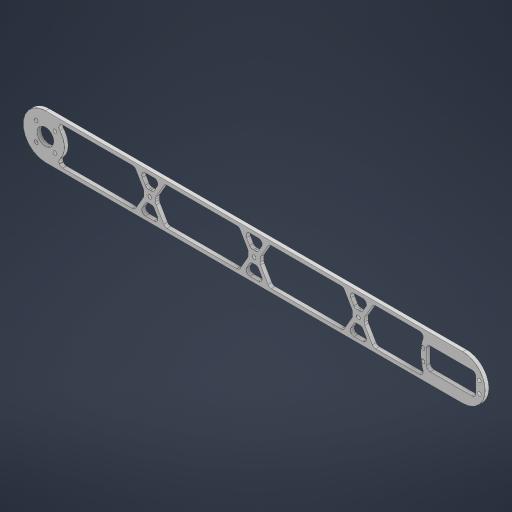
# Autodesk Inventor part: Arm3rdLinkServo
Saved by Autodesk Inventor 2023 (Build 270158000, 158)
## iProperties
Created: 2023-12-24
Part Number: Arm3rdLinkServo
Material: Generic
Document SubType Name: Modeling
Designer: kelle
Density: 1 g/cm^3
Appearance: Default
Author: kelle
Autodesk Inventor part; units mm, degrees
ref_plane "YZ Plane" through (0, 0, 0) normal (1, 0, 0) x (0, 1, 0)
ref_plane "XZ Plane" through (0, 0, 0) normal (0, 1, 0) x (-1, 0, 0)
ref_plane "XY Plane" through (0, 0, 0) normal (0, 0, 1) x (1, 0, 0)
sketch "Sketch1" plane through (0, 0, 0) normal (0, 0, 1) x (1, 0, 0)
  line L0 (177.8, 0) -> (-177.8, 0) construction
  line L1 (177.8, 19.05) -> (-177.8, 19.05)
  line L2 (-177.8, -19.05) -> (177.8, -19.05)
  arc A0 (177.8, -19.05) -> (177.8, 19.05) centre (177.8, 0) ccw
  arc A1 (-177.8, 19.05) -> (-177.8, -19.05) centre (-177.8, 0) ccw
  circle A2 centre (-177.8, 0) radius 7
  line L3 (-185.8, -8) -> (-169.8, -8) construction
  line L4 (-169.8, -8) -> (-169.8, 8) construction
  line L5 (-169.8, 8) -> (-185.8, 8) construction
  line L6 (-185.8, 8) -> (-185.8, -8) construction
  line L7 (-185.8, -8) -> (-169.8, 8) construction
  line L8 (-169.8, -8) -> (-185.8, 8) construction
  circle A3 centre (-185.8, 8) radius 1.5875
  circle A4 centre (-169.8, 8) radius 1.5875
  circle A5 centre (-185.8, -8) radius 1.5875
  circle A6 centre (-169.8, -8) radius 1.5875
  circle A7 centre (0, 0) radius 2
  circle A8 centre (-88.9, 0) radius 2
  circle A9 centre (88.9, 0) radius 2
  circle A10 centre (0, 0) radius 2
  circle A11 centre (177.8, 0) radius 3
  line L9 (177.8, 0) -> (192, 0) construction
  line L10 (192, 0) -> (192, 4.95) construction
  circle A12 centre (192, 4.95) radius 1.5875
  circle A13 centre (144, 4.95) radius 1.5875
  circle A14 centre (192, -4.95) radius 1.5875
  circle A15 centre (144, -4.95) radius 1.5875
  line L11 (192, 4.95) -> (189, 4.95) construction
  line L12 (189, 9.525) -> (147, 9.525)
  line L13 (147, 9.525) -> (147, -9.525)
  line L14 (189, -9.525) -> (189, 9.525)
  line L15 (147, -9.525) -> (189, -9.525)
  dimension "d0" = 177.8
  dimension "d1" = 38.1
  dimension "d2" = 14
  dimension "d3" = 16
  dimension "d4" = 16
  dimension "d5" = 3.175
  dimension "d8" = 16
  dimension "d11" = 16
  dimension "d14" = 4
  dimension "d17" = 88.9
  dimension "d20" = 88.9
  dimension "d23" = 6
  dimension "d24" = 14.2
  dimension "d25" = 4.95
  dimension "d27" = 3.175
  dimension "d31" = 48
  dimension "d34" = 9.9
  dimension "d37" = 3
  dimension "d38" = 42
  dimension "d39" = 9.525
  dimension "d40" = 19.05
  dimension "d41" = 42
  dimension "d60" = 3
  constraints: 34 end point, 16 centre point, 9 horizontal, 5 coincident, 4 point on circle, 4 tangent, 4 vertical, 3 midpoint, 3 parallel, 1 perpendicular, 18 other
  measures "d0" distance of point (0, 0) L0.end
  measures "d1" diameter of A1
  measures "d2" diameter of A2
  measures "d3" distance of L3.start L3.end
  measures "d4" distance of L4.end L3.end
  measures "d5" diameter of A3
  measures "d8" distance of A3.centre A4.centre
  measures "d11" distance of A3.centre A5.centre
  measures "d14" diameter of A7
  measures "d17" distance of A7.centre A8.centre
  measures "d20" distance of A7.centre A9.centre
  measures "d23" diameter of A11
  measures "d24" distance of L9.start L9.end
  measures "d25" distance of L9.end L10.end
  measures "d27" diameter of A12
  measures "d31" distance of L11.start A13.centre
  measures "d34" distance of L11.start A14.centre
  measures "d37" distance of L11.start L11.end
  measures "d38" distance of L12.start L12.end
  measures "d39" distance between parallel lines of L12 L0
  measures "d40" distance of L12.end L13.end
  measures "d41" distance of L13.end L14.start
  measures "d60" distance from line of L10.end L14
extrude "Extrusion1" add sketch "Sketch1" along normal blind 3.175 contours A0 L2 A1 L1
sketch "Sketch4" plane through (0, 0, 3.175) normal (0, 0, 1) x (1, 0, 0)
  arc A0 (-177.8, 19.05) -> (-177.8, -19.05) centre (-177.8, 0) ccw
  line L0 (-177.8, -19.05) -> (177.8, -19.05)
  arc A1 (177.8, -19.05) -> (177.8, 19.05) centre (177.8, 0) ccw
  line L1 (177.8, 19.05) -> (-177.8, 19.05)
  circle A2 centre (0, 0) radius 2
  circle A3 centre (-88.9, 0) radius 2
  circle A4 centre (88.9, 0) radius 2
  circle A5 centre (144, 4.95) radius 1.5875
  circle A6 centre (144, -4.95) radius 1.5875
  line L2 (189, 9.525) -> (189, -9.525)
  line L3 (189, -9.525) -> (147, -9.525)
  line L4 (147, -9.525) -> (147, 9.525)
  line L5 (147, 9.525) -> (189, 9.525)
  circle A7 centre (192, -4.95) radius 1.5875
  circle A8 centre (192, 4.95) radius 1.5875
  circle A9 centre (-169.8, -8) radius 1.5875
  circle A10 centre (-185.8, -8) radius 1.5875
  circle A11 centre (-169.8, 8) radius 1.5875
  circle A12 centre (-185.8, 8) radius 1.5875
  circle A13 centre (-177.8, 0) radius 7
  circle A14 centre (-177.8, 0) radius 7 construction
  circle A15 centre (-177.8, 0) radius 12.901208 construction
  circle A16 centre (-177.8, 0) radius 16.076208
  circle A17 centre (-88.9, 0) radius 5.175
  circle A18 centre (0, 0) radius 5.175
  circle A19 centre (88.9, 0) radius 5.175
  circle A20 centre (177.8, 0) radius 35.74804
  circle A21 centre (144, -4.95) radius 1.5875 construction
  circle A22 centre (177.8, 0) radius 38.92304 construction
  line L6 (-177.8, 0) -> (-133.35, 0) construction
  line L7 (-177.8, 0) -> (-133.35, 0) construction
  line L8 (-177.8, 0) -> (-155.575, 38.494829)
  line L9 (-155.575, 38.494829) -> (-111.125, 38.494829)
  line L10 (-111.125, 38.494829) -> (-88.9, 0)
  line L11 (-88.9, 0) -> (-111.125, -38.494829)
  line L12 (-111.125, -38.494829) -> (-155.575, -38.494829)
  line L13 (-155.575, -38.494829) -> (-177.8, 0)
  arc A23 (-177.8, 15.875) -> (-177.8, -15.875) centre (-177.8, 0) ccw
  line L14 (-177.8, -15.875) -> (177.8, -15.875)
  arc A24 (177.8, -15.875) -> (177.8, 15.875) centre (177.8, 0) ccw
  line L15 (177.8, 15.875) -> (-177.8, 15.875)
  line L16 (-112.958087, 35.319829) -> (-153.741913, 35.319829)
  line L17 (-153.741913, 35.319829) -> (-174.133826, 0)
  line L18 (-174.133826, 0) -> (-153.741913, -35.319829)
  line L19 (-153.741913, -35.319829) -> (-112.958087, -35.319829)
  line L20 (-112.958087, -35.319829) -> (-92.566174, 0)
  line L21 (-92.566174, 0) -> (-112.958087, 35.319829)
  line L22 (177.8, 19.05) -> (-177.8, 19.05) construction
  line L23 (-88.9, 19.05) -> (-88.9, -19.05) construction
  line L24 (0, 19.05) -> (0, -19.05) construction
  line L25 (0, 0) -> (-22.225, 38.494829)
  line L26 (-66.675, 38.494829) -> (-88.9, 0)
  line L27 (-88.9, 0) -> (-66.675, -38.494829)
  line L28 (-22.225, -38.494829) -> (0, 0)
  line L29 (-24.058087, 35.319829) -> (-3.666174, 0)
  line L30 (-3.666174, 0) -> (-24.058087, -35.319829)
  line L31 (-64.841913, -35.319829) -> (-85.233826, 0)
  line L32 (-85.233826, 0) -> (-64.841913, 35.319829)
  line L33 (177.8, 0) -> (155.575, 38.494829)
  line L34 (111.125, 38.494829) -> (88.9, 0)
  line L35 (88.9, 0) -> (111.125, -38.494829)
  line L36 (155.575, -38.494829) -> (177.8, 0)
  line L37 (153.741913, 35.319829) -> (174.133826, 0)
  line L38 (174.133826, 0) -> (153.741913, -35.319829)
  line L39 (112.958087, -35.319829) -> (92.566174, 0)
  line L40 (92.566174, 0) -> (112.958087, 35.319829)
  line L41 (0, 0) -> (22.225, 38.494829)
  line L42 (24.058087, 35.319829) -> (3.666174, 0)
  line L43 (3.666174, 0) -> (24.058087, -35.319829)
  line L44 (22.225, -38.494829) -> (0, 0)
  line L45 (64.841913, -35.319829) -> (85.233826, 0)
  line L46 (88.9, 0) -> (66.675, -38.494829)
  line L47 (85.233826, 0) -> (64.841913, 35.319829)
  line L48 (66.675, 38.494829) -> (88.9, 0)
  point P0 (79.734564, 15.875)
  point P1 (86.3125, 4.481681)
  point P2 (91.4875, 4.481681)
  point P3 (98.065436, 15.875)
  point P4 (98.065436, -15.875)
  point P5 (91.4875, -4.481681)
  point P6 (86.3125, -4.481681)
  point P7 (79.734564, -15.875)
  point P8 (2.5875, 4.481681)
  point P9 (9.165436, 15.875)
  point P10 (-9.165436, 15.875)
  point P11 (-2.5875, 4.481681)
  point P12 (9.165436, -15.875)
  point P13 (2.5875, -4.481681)
  point P14 (-2.5875, -4.481681)
  point P15 (-9.165436, -15.875)
  point P16 (-79.734564, -15.875)
  point P17 (-86.3125, -4.481681)
  point P18 (-91.4875, -4.481681)
  point P19 (-98.065436, -15.875)
  point P20 (-86.3125, 4.481681)
  point P21 (-79.734564, 15.875)
  point P22 (-98.065436, 15.875)
  point P23 (-91.4875, 4.481681)
  point P24 (93.692912, -1.951568)
  point P25 (101.73161, -15.875)
  point P26 (145.770221, -15.875)
  point P27 (145.770221, 15.875)
  point P28 (101.73161, 15.875)
  point P29 (93.692912, 1.951568)
  point P30 (76.06839, -15.875)
  point P31 (84.107088, -1.951568)
  point P32 (84.107088, 1.951568)
  point P33 (76.06839, 15.875)
  point P34 (12.83161, 15.875)
  point P35 (4.792912, 1.951568)
  point P36 (4.792912, -1.951568)
  point P37 (12.83161, -15.875)
  point P38 (-76.06839, 15.875)
  point P39 (-84.107088, 1.951568)
  point P40 (-84.107088, -1.951568)
  point P41 (-76.06839, -15.875)
  point P42 (-12.83161, -15.875)
  point P43 (-4.792912, -1.951568)
  point P44 (-4.792912, 1.951568)
  point P45 (-12.83161, 15.875)
  point P46 (-93.692912, 1.951568)
  point P47 (-101.73161, 15.875)
  point P48 (-164.96839, 15.875)
  point P49 (-167.170587, 12.060683)
  point P50 (-167.170587, -12.060683)
  point P51 (-164.96839, -15.875)
  point P52 (-101.73161, -15.875)
  point P53 (-93.692912, -1.951568)
  dimension "d61" = 3.175
  dimension "d62" = 3.175
  dimension "d63" = 3.175
  dimension "d64" = 3.175
  dimension "d65" = 3.175
  dimension "d66" = 44.45
  dimension "d67" = 0
  dimension "d68" = 3.175
  dimension "d69" = 3.175
  constraints: 84 end point, 33 symmetric about line, 9 centre point, 4 point on circle, 3 coincident, 2 horizontal, 2 midpoint, 2 point on line, 2 tangent, 1 collinear, 1 perpendicular, 21 other
  measures "d61" radial gap between concentric circles of A15 A16
  measures "d62" radial gap between concentric circles of A3 A17
  measures "d63" radial gap between concentric circles of A2 A18
  measures "d64" radial gap between concentric circles of A4 A19
  measures "d65" radial gap between concentric circles of A20 A22
  measures "d66" distance of L6.start L6.end
  measures "d67" distance between parallel lines of L6 L7
  measures "d68" distance between parallel lines of L1 L15
  measures "d69" distance between parallel lines of L9 L16
extrude "Extrusion4" cut sketch "Sketch4" against normal through all contours L15 L21 A17 L20 L14 L18 A16 L17 | L15 L26 A17 L10 | L11 A17 L27 L14 | L15 L29 A18 L30 L14 L31 A17 L32 | L15 L41 A18 L25 | L28 A18 L44 L14 | L15 L47 A19 L45 L14 L43 A18 L42 | L15 L34 A19 L48 | L46 A19 L35 L14 | L15 A20 L14 L39 A19 L40
fillet "Fillet2" radius 3.175 58 edges at (-86.3125, -4.4817, 1.5875) (-79.7346, -15.875, 1.5875) (-91.4875, -4.4817, 1.5875) (-98.0654, -15.875, 1.5875) (2.5875, -4.4817, 1.5875) (9.1654, -15.875, 1.5875) (-2.5875, -4.4817, 1.5875) (-9.1654, -15.875, 1.5875) (-101.7316, 15.875, 1.5875) (-93.6929, 1.9516, 1.5875) (-164.9684, 15.875, 1.5875) (-167.1706, 12.0607, 1.5875) (-167.1706, -12.0607, 1.5875) (-164.9684, -15.875, 1.5875) (-101.7316, -15.875, 1.5875) (-93.6929, -1.9516, 1.5875) (-84.1071, 1.9516, 1.5875) (-76.0684, 15.875, 1.5875) (-84.1071, -1.9516, 1.5875) (-76.0684, -15.875, 1.5875) (-12.8316, -15.875, 1.5875) (-4.7929, -1.9516, 1.5875) (-4.7929, 1.9516, 1.5875) (-12.8316, 15.875, 1.5875) (91.4875, -4.4817, 1.5875) (98.0654, -15.875, 1.5875) (86.3125, -4.4817, 1.5875) (79.7346, -15.875, 1.5875) (84.1071, -1.9516, 1.5875) (76.0684, -15.875, 1.5875) (84.1071, 1.9516, 1.5875) (76.0684, 15.875, 1.5875) (12.8316, 15.875, 1.5875) (4.7929, 1.9516, 1.5875) (4.7929, -1.9516, 1.5875) (12.8316, -15.875, 1.5875) (189, 9.525, 1.5875) (189, -9.525, 1.5875) (147, 9.525, 1.5875) (147, -9.525, 1.5875) (-79.7346, 15.875, 1.5875) (-86.3125, 4.4817, 1.5875) (-98.0654, 15.875, 1.5875) (-91.4875, 4.4817, 1.5875) (9.1654, 15.875, 1.5875) (2.5875, 4.4817, 1.5875) (-9.1654, 15.875, 1.5875) (-2.5875, 4.4817, 1.5875) (145.7702, 15.875, 1.5875) (101.7316, 15.875, 1.5875) (93.6929, 1.9516, 1.5875) (93.6929, -1.9516, 1.5875) (101.7316, -15.875, 1.5875) (145.7702, -15.875, 1.5875) (86.3125, 4.4817, 1.5875) (79.7346, 15.875, 1.5875) (91.4875, 4.4817, 1.5875) (98.0654, 15.875, 1.5875)
sketch "Sketch5" plane through (0, 0, 3.175) normal (0, 0, 1) x (1, 0, 0)
  circle A0 centre (-177.8, 0) radius 7
  circle A1 centre (-185.8, 8) radius 1.5875
  circle A2 centre (-169.8, 8) radius 1.5875
  circle A3 centre (-185.8, -8) radius 1.5875
  circle A4 centre (-169.8, -8) radius 1.5875
  circle A5 centre (192, 4.95) radius 1.5875
  circle A6 centre (192, -4.95) radius 1.5875
  line L0 (189, 6.35) -> (189, -6.35)
  arc A7 (185.825, -9.525) -> (189, -6.35) centre (185.825, -6.35) ccw
  line L1 (185.825, -9.525) -> (150.175, -9.525)
  arc A8 (147, -6.35) -> (150.175, -9.525) centre (150.175, -6.35) ccw
  line L2 (147, -6.35) -> (147, 6.35)
  arc A9 (150.175, 9.525) -> (147, 6.35) centre (150.175, 6.35) ccw
  line L3 (150.175, 9.525) -> (185.825, 9.525)
  arc A10 (189, 6.35) -> (185.825, 9.525) centre (185.825, 6.35) ccw
  circle A11 centre (144, 4.95) radius 1.5875
  arc A12 (142.429255, 5.180035) -> (142.429255, -5.180035) centre (177.8, 0) ccw
  circle A13 centre (144, -4.95) radius 1.5875
  arc A14 (142.429255, -5.180035) -> (144.008397, -11.664045) centre (177.8, 0) ccw
  arc A15 (141.00716, -15.875) -> (144.008397, -11.664045) centre (141.00716, -12.7) ccw
  line L4 (141.00716, -15.875) -> (103.564697, -15.875)
  arc A16 (100.815066, -14.2875) -> (103.564697, -15.875) centre (103.564697, -12.7) ccw
  line L5 (100.815066, -14.2875) -> (94.360719, -3.108243)
  arc A17 (93.98845, -0.942496) -> (94.360719, -3.108243) centre (97.11035, -1.520743) ccw
  arc A18 (93.98845, -0.942496) -> (93.98845, 0.942496) centre (88.9, 0) ccw
  arc A19 (94.360719, 3.108243) -> (93.98845, 0.942496) centre (97.11035, 1.520743) ccw
  line L6 (94.360719, 3.108243) -> (100.815066, 14.2875)
  arc A20 (103.564697, 15.875) -> (100.815066, 14.2875) centre (103.564697, 12.7) ccw
  line L7 (103.564697, 15.875) -> (141.00716, 15.875)
  arc A21 (144.008397, 11.664045) -> (141.00716, 15.875) centre (141.00716, 12.7) ccw
  arc A22 (144.008397, 11.664045) -> (142.429255, 5.180035) centre (177.8, 0) ccw
  circle A23 centre (88.9, 0) radius 2
  circle A24 centre (-88.9, 0) radius 2
  circle A25 centre (0, 0) radius 2
  arc A26 (-177.8, 19.05) -> (-177.8, -19.05) centre (-177.8, 0) ccw
  line L8 (-177.8, -19.05) -> (177.8, -19.05)
  arc A27 (177.8, -19.05) -> (177.8, 19.05) centre (177.8, 0) ccw
  line L9 (177.8, 19.05) -> (-177.8, 19.05)
  line L10 (-165.963476, 14.151461) -> (-165.884934, 14.2875)
  arc A28 (-163.135303, 15.875) -> (-165.884934, 14.2875) centre (-163.135303, 12.7) ccw
  line L11 (-163.135303, 15.875) -> (-103.564697, 15.875)
  arc A29 (-100.815066, 14.2875) -> (-103.564697, 15.875) centre (-103.564697, 12.7) ccw
  line L12 (-100.815066, 14.2875) -> (-94.360719, 3.108243)
  arc A30 (-93.98845, 0.942496) -> (-94.360719, 3.108243) centre (-97.11035, 1.520743) ccw
  arc A31 (-93.98845, 0.942496) -> (-93.98845, -0.942496) centre (-88.9, 0) ccw
  arc A32 (-94.360719, -3.108243) -> (-93.98845, -0.942496) centre (-97.11035, -1.520743) ccw
  line L13 (-94.360719, -3.108243) -> (-100.815066, -14.2875)
  arc A33 (-103.564697, -15.875) -> (-100.815066, -14.2875) centre (-103.564697, -12.7) ccw
  line L14 (-103.564697, -15.875) -> (-163.135303, -15.875)
  arc A34 (-165.884934, -14.2875) -> (-163.135303, -15.875) centre (-163.135303, -12.7) ccw
  line L15 (-165.884934, -14.2875) -> (-165.963476, -14.151461)
  arc A35 (-165.619463, -10.491853) -> (-165.963476, -14.151461) centre (-163.213845, -12.563961) ccw
  arc A36 (-165.619463, -10.491853) -> (-165.619463, 10.491853) centre (-177.8, 0) ccw
  arc A37 (-165.963476, 14.151461) -> (-165.619463, 10.491853) centre (-163.213845, 12.563961) ccw
  line L16 (-92.761408, 6.688154) -> (-95.315805, 11.1125)
  arc A38 (-92.566174, 15.875) -> (-95.315805, 11.1125) centre (-92.566174, 12.7) ccw
  line L17 (-92.566174, 15.875) -> (-85.233826, 15.875)
  arc A39 (-82.484195, 11.1125) -> (-85.233826, 15.875) centre (-85.233826, 12.7) ccw
  line L18 (-82.484195, 11.1125) -> (-85.038592, 6.688154)
  arc A40 (-88.210965, 5.128923) -> (-85.038592, 6.688154) centre (-87.788223, 8.275654) ccw
  arc A41 (-88.210965, 5.128923) -> (-89.589035, 5.128923) centre (-88.9, 0) ccw
  arc A42 (-92.761408, 6.688154) -> (-89.589035, 5.128923) centre (-90.011777, 8.275654) ccw
  line L19 (82.484195, -11.1125) -> (85.038592, -6.688154)
  arc A43 (88.210965, -5.128923) -> (85.038592, -6.688154) centre (87.788223, -8.275654) ccw
  arc A44 (88.210965, -5.128923) -> (89.589035, -5.128923) centre (88.9, 0) ccw
  arc A45 (92.761408, -6.688154) -> (89.589035, -5.128923) centre (90.011777, -8.275654) ccw
  line L20 (92.761408, -6.688154) -> (95.315805, -11.1125)
  arc A46 (92.566174, -15.875) -> (95.315805, -11.1125) centre (92.566174, -12.7) ccw
  line L21 (92.566174, -15.875) -> (85.233826, -15.875)
  arc A47 (82.484195, -11.1125) -> (85.233826, -15.875) centre (85.233826, -12.7) ccw
  line L22 (-3.861408, 6.688154) -> (-6.415805, 11.1125)
  arc A48 (-3.666174, 15.875) -> (-6.415805, 11.1125) centre (-3.666174, 12.7) ccw
  line L23 (-3.666174, 15.875) -> (3.666174, 15.875)
  arc A49 (6.415805, 11.1125) -> (3.666174, 15.875) centre (3.666174, 12.7) ccw
  line L24 (6.415805, 11.1125) -> (3.861408, 6.688154)
  arc A50 (0.689035, 5.128923) -> (3.861408, 6.688154) centre (1.111777, 8.275654) ccw
  arc A51 (0.689035, 5.128923) -> (-0.689035, 5.128923) centre (0, 0) ccw
  arc A52 (-3.861408, 6.688154) -> (-0.689035, 5.128923) centre (-1.111777, 8.275654) ccw
  line L25 (-76.984934, -14.2875) -> (-83.439281, -3.108243)
  arc A53 (-83.81155, -0.942496) -> (-83.439281, -3.108243) centre (-80.68965, -1.520743) ccw
  arc A54 (-83.81155, -0.942496) -> (-83.81155, 0.942496) centre (-88.9, 0) ccw
  arc A55 (-83.439281, 3.108243) -> (-83.81155, 0.942496) centre (-80.68965, 1.520743) ccw
  line L26 (-83.439281, 3.108243) -> (-76.984934, 14.2875)
  arc A56 (-74.235303, 15.875) -> (-76.984934, 14.2875) centre (-74.235303, 12.7) ccw
  line L27 (-74.235303, 15.875) -> (-14.664697, 15.875)
  arc A57 (-11.915066, 14.2875) -> (-14.664697, 15.875) centre (-14.664697, 12.7) ccw
  line L28 (-11.915066, 14.2875) -> (-5.460719, 3.108243)
  arc A58 (-5.08845, 0.942496) -> (-5.460719, 3.108243) centre (-8.21035, 1.520743) ccw
  arc A59 (-5.08845, 0.942496) -> (-5.08845, -0.942496) centre (0, 0) ccw
  arc A60 (-5.460719, -3.108243) -> (-5.08845, -0.942496) centre (-8.21035, -1.520743) ccw
  line L29 (-5.460719, -3.108243) -> (-11.915066, -14.2875)
  arc A61 (-14.664697, -15.875) -> (-11.915066, -14.2875) centre (-14.664697, -12.7) ccw
  line L30 (-14.664697, -15.875) -> (-74.235303, -15.875)
  arc A62 (-76.984934, -14.2875) -> (-74.235303, -15.875) centre (-74.235303, -12.7) ccw
  line L31 (-95.315805, -11.1125) -> (-92.761408, -6.688154)
  arc A63 (-89.589035, -5.128923) -> (-92.761408, -6.688154) centre (-90.011777, -8.275654) ccw
  arc A64 (-89.589035, -5.128923) -> (-88.210965, -5.128923) centre (-88.9, 0) ccw
  arc A65 (-85.038592, -6.688154) -> (-88.210965, -5.128923) centre (-87.788223, -8.275654) ccw
  line L32 (-85.038592, -6.688154) -> (-82.484195, -11.1125)
  arc A66 (-85.233826, -15.875) -> (-82.484195, -11.1125) centre (-85.233826, -12.7) ccw
  line L33 (-85.233826, -15.875) -> (-92.566174, -15.875)
  arc A67 (-95.315805, -11.1125) -> (-92.566174, -15.875) centre (-92.566174, -12.7) ccw
  line L34 (95.315805, 11.1125) -> (92.761408, 6.688154)
  arc A68 (89.589035, 5.128923) -> (92.761408, 6.688154) centre (90.011777, 8.275654) ccw
  arc A69 (89.589035, 5.128923) -> (88.210965, 5.128923) centre (88.9, 0) ccw
  arc A70 (85.038592, 6.688154) -> (88.210965, 5.128923) centre (87.788223, 8.275654) ccw
  line L35 (85.038592, 6.688154) -> (82.484195, 11.1125)
  arc A71 (85.233826, 15.875) -> (82.484195, 11.1125) centre (85.233826, 12.7) ccw
  line L36 (85.233826, 15.875) -> (92.566174, 15.875)
  arc A72 (95.315805, 11.1125) -> (92.566174, 15.875) centre (92.566174, 12.7) ccw
  line L37 (-6.415805, -11.1125) -> (-3.861408, -6.688154)
  arc A73 (-0.689035, -5.128923) -> (-3.861408, -6.688154) centre (-1.111777, -8.275654) ccw
  arc A74 (-0.689035, -5.128923) -> (0.689035, -5.128923) centre (0, 0) ccw
  arc A75 (3.861408, -6.688154) -> (0.689035, -5.128923) centre (1.111777, -8.275654) ccw
  line L38 (3.861408, -6.688154) -> (6.415805, -11.1125)
  arc A76 (3.666174, -15.875) -> (6.415805, -11.1125) centre (3.666174, -12.7) ccw
  line L39 (3.666174, -15.875) -> (-3.666174, -15.875)
  arc A77 (-6.415805, -11.1125) -> (-3.666174, -15.875) centre (-3.666174, -12.7) ccw
  line L40 (76.984934, 14.2875) -> (83.439281, 3.108243)
  arc A78 (83.81155, 0.942496) -> (83.439281, 3.108243) centre (80.68965, 1.520743) ccw
  arc A79 (83.81155, 0.942496) -> (83.81155, -0.942496) centre (88.9, 0) ccw
  arc A80 (83.439281, -3.108243) -> (83.81155, -0.942496) centre (80.68965, -1.520743) ccw
  line L41 (83.439281, -3.108243) -> (76.984934, -14.2875)
  arc A81 (74.235303, -15.875) -> (76.984934, -14.2875) centre (74.235303, -12.7) ccw
  line L42 (74.235303, -15.875) -> (14.664697, -15.875)
  arc A82 (11.915066, -14.2875) -> (14.664697, -15.875) centre (14.664697, -12.7) ccw
  line L43 (11.915066, -14.2875) -> (5.460719, -3.108243)
  arc A83 (5.08845, -0.942496) -> (5.460719, -3.108243) centre (8.21035, -1.520743) ccw
  arc A84 (5.08845, -0.942496) -> (5.08845, 0.942496) centre (0, 0) ccw
  arc A85 (5.460719, 3.108243) -> (5.08845, 0.942496) centre (8.21035, 1.520743) ccw
  line L44 (5.460719, 3.108243) -> (11.915066, 14.2875)
  arc A86 (14.664697, 15.875) -> (11.915066, 14.2875) centre (14.664697, 12.7) ccw
  line L45 (14.664697, 15.875) -> (74.235303, 15.875)
  arc A87 (76.984934, 14.2875) -> (74.235303, 15.875) centre (74.235303, 12.7) ccw
  circle A88 centre (-88.9, 0) radius 2
  circle A89 centre (-88.9, 0) radius 1.5875
  circle A90 centre (0, 0) radius 1.5875
  circle A91 centre (88.9, 0) radius 1.5875
  dimension "d73" = 3.175
  dimension "d74" = 3.175
  dimension "d75" = 3.175
  constraints: 3 centre point, 3 coincident, 2 other
  measures "d73" diameter of A89
  measures "d74" diameter of A90
  measures "d75" diameter of A91
extrude "Extrusion5" add sketch "Sketch5" against normal blind 3.175 contours A23 | A24 | A25
body "Solid1"
